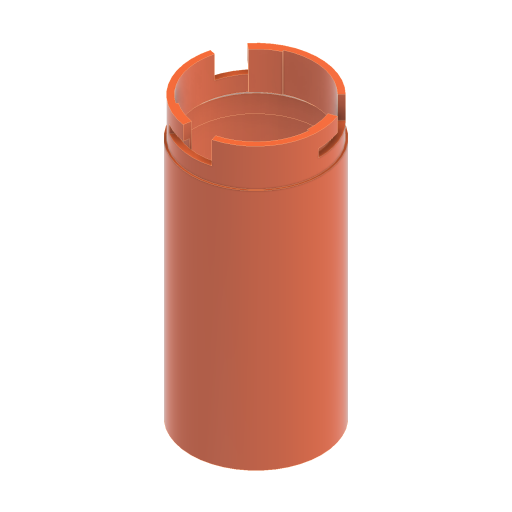
# Autodesk Inventor part: Lower skin
Saved by Autodesk Inventor 2024 (Build 280153000, 153)
## iProperties
Created: 2023-12-30
Part Number: Lower skin
Material: Plastic, Opaque White
Document SubType Name: Modeling
Designer: Jamie
Density: 0.952 g/cm^3
Appearance: Smooth - Light Orange
Author: Jamie
Autodesk Inventor part; units mm, degrees
sketch "Sketch1" plane through (0, 0, 0) normal (0, 1, 0) x (-1, 0, 0)
  circle A0 centre (0, 0) radius 35
  circle A1 centre (0, 0) radius 34.5
  dimension "d0" = 70
  dimension "d1" = 69
  constraints: 2 centre point, 2 coincident
  measures "d0" diameter of A0
  measures "d1" diameter of A1
extrude "Extrusion1" add sketch "Sketch1" along normal blind 130
ref_plane "Work Plane2" through (35, 0, 0) normal (1, 0, 0) x (0, 1, 0)
sketch "Sketch5" plane through (0, 130, 0) normal (0, 1, 0) x (1, 0, 0)
  circle A0 centre (0, 0) radius 34
  circle A1 centre (0, 0) radius 31
  dimension "d44" = 68
  dimension "d45" = 62
  constraints: 2 centre point, 2 coincident
  measures "d44" diameter of A0
  measures "d45" diameter of A1
extrude "Extrusion3" add sketch "Sketch5" along normal blind 20
sketch "Sketch6" plane through (0, 130, 0) normal (0, -1, 0) x (1, 0, 0)
  circle A0 centre (0, 0) radius 33.5
  circle A1 centre (0, 0) radius 34.5 projected
  circle A2 centre (0, 0) radius 35
  constraints: 2 centre point, 2 coincident
extrude "Extrusion4" add sketch "Sketch6" along normal blind 12.5 contours A1
ref_plane "Work Plane4" through (34, 0, 0) normal (1, 0, 0) x (0, 1, 0)
ref_plane "Work Plane5" through (0, 8, 0) normal (0, -1, 0) x (1, 0, 0)
sketch "Sketch9" plane through (0, 8, 0) normal (0, -1, 0) x (1, 0, 0)
  line L0 (0, 0) -> (34.5, 0) construction
  circle A0 centre (0, 0) radius 34.5 construction
  line L1 (0, 0) -> (32.4194, -11.7997) construction
  arc A1 (29.6003, -10.7736) -> (31.5, 0) centre (0, 0) ccw
  arc A2 (32.4194, -11.7997) -> (34.5, 0) centre (0, 0) ccw
  line L2 (34.5, 0) -> (31.5, 0)
  line L3 (29.6003, -10.7736) -> (32.4194, -11.7997)
  dimension "d75" = 20
  dimension "d76" = 31.5
  dimension "d85" = 69
  constraints: 8 end point, 6 point on circle, 2 centre point, 2 coincident, 2 point on line, 1 horizontal
  measures "d75" angle of L1 L0
  measures "d76" radius of A1
  measures "d85" diameter of A0
extrude "Extrusion5" add sketch "Sketch9" against normal blind 4
chamfer "Chamfer1" distance 1.5 angle 60 2 edges at (33, 8, 0) (31.0099, 8, -11.2867) measured on face at (32.8292, 8, -6.4086)
ref_plane "Work Plane6" through (0, 142.25, 0) normal (0, 1, 0) x (1, 0, 0)
sketch "Sketch10" plane through (0, 142.25, 0) normal (0, 1, 0) x (1, 0, 0)
  line L0 (0, 0) -> (37.2135, -0.3248)
  line L1 (0, 0) -> (36.1959, 0) construction
  line L2 (0, 0) -> (35.6152, 13.316)
  line L3 (35.6152, 13.316) -> (37.2135, -0.3248)
  dimension "d87" = 0.5
  dimension "d88" = 21
  constraints: 8 end point, 1 horizontal
  measures "d87" angle of L1 L0
  measures "d88" angle of L2 L0
extrude "Extrusion6" cut sketch "Sketch10" against normal blind 4.5
sketch "Sketch11" plane through (0, 137.75, 0) normal (0, 1, 0) x (1, 0, 0)
  arc A0 (30.9988, -0.2705) -> (29.0368, 10.8564) centre (0, 0) ccw projected
  line L0 (0, 0) -> (29.0368, 10.8564)
  line L1 (29.0368, 10.8564) -> (36.6215, 13.6922)
  line L2 (36.6215, 13.6922) -> (28.642, 29.1463)
  line L3 (28.642, 29.1463) -> (0, 0)
  dimension "d91" = 25
  constraints: 8 end point
  measures "d91" angle of L0 L3
extrude "Extrusion7" cut sketch "Sketch11" along normal through all
sketch "Sketch12" plane through (0, 130, 0) normal (0, -1, 0) x (1, 0, 0)
  line L0 (0, 0) -> (36.23, 0) construction
  line L1 (0, 0) -> (37.1898, 2.9269) construction
  line L2 (0, 0) -> (35.2666, -13.1857) construction
  arc A0 (29.0368, -10.8564) -> (30.9044, 2.4322) centre (0, 0) ccw
  arc A1 (28.1002, -10.5062) -> (29.9075, 2.3538) centre (0, 0) ccw
  line L3 (30.9044, 2.4322) -> (29.9075, 2.3538)
  line L4 (29.0368, -10.8564) -> (28.1002, -10.5062)
  dimension "d94" = 4.5
  dimension "d95" = 20.5
  dimension "d96" = 31
  dimension "d97" = 30
  constraints: 10 end point, 4 point on circle, 4 point on line, 2 centre point, 2 coincident, 2 collinear, 1 horizontal
  measures "d94" angle of L0 L1
  measures "d95" angle of L2 L0
  measures "d96" radius of A0
  measures "d97" radius of A1
extrude "Extrusion8" add sketch "Sketch12" against normal blind 20
pattern_circular "Circular Pattern4" count 3 over 360 about axis through (0, 0, 0) along (0, 1, 0) of "Extrusion6", "Extrusion7", "Extrusion8"
chamfer "Chamfer2" distance 3 angle 45 1 edges at (-33.5, 130, 0)
pattern_circular "Circular Pattern5" count 3 over 360 about axis through (0, 0, 0) along (0, 1, 0) of "Extrusion5", "Chamfer1"
body "Solid1"
